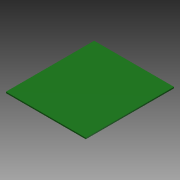
# Autodesk Inventor part: Dish_Board
Saved by Autodesk Inventor 2014 (Build 180170000, 170)
## iProperties
Created: 2015-01-07
Part Number: Dish_Board
Material: Generic
Document SubType Name: Modeling
Designer: Owner
Density: 1 g/cm^3
Appearance: Smooth - Dark Forest Green
Author: Owner
Autodesk Inventor part; units mm, degrees
ref_plane "YZ Plane" through (0, 0, 0) normal (1, 0, 0) x (0, 1, 0)
ref_plane "XZ Plane" through (0, 0, 0) normal (0, 1, 0) x (-1, 0, 0)
ref_plane "XY Plane" through (0, 0, 0) normal (0, 0, 1) x (1, 0, 0)
sketch "Sketch1" plane through (0, 0, 0) normal (0, 1, 0) x (-1, 0, 0)
  line L0 (-12.7166, 29.9631) -> (89.1374, 29.9631)
  line L1 (89.1374, 29.9631) -> (89.1374, -82.5589)
  line L2 (89.1374, -82.5589) -> (-12.7166, -82.5589)
  line L3 (-12.7166, -82.5589) -> (-12.7166, 29.9631)
  point P0 (0, 0)
  dimension "d0" = 101.854
  dimension "d1" = 112.522
  constraints: 8 end point, 2 parallel, 1 horizontal, 1 perpendicular
  measures "d0" distance of L0.start L0.end
  measures "d1" distance of L0.end L1.end
extrude "Extrusion1" add sketch "Sketch1" along normal blind 1.6
body "Solid1"
